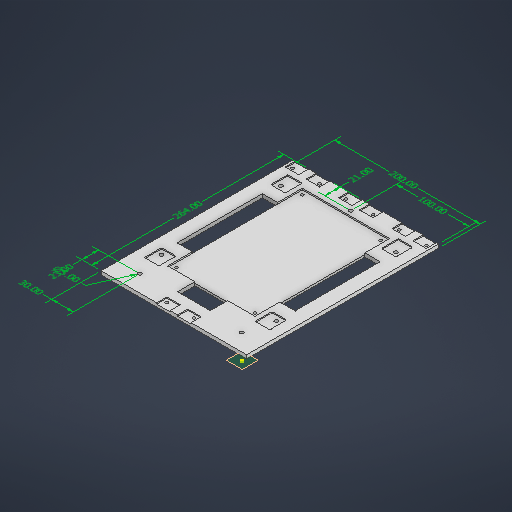
# Autodesk Inventor part: RobotPCBLevel
Saved by Autodesk Inventor 2026 (Build 300175000, 175)
## iProperties
Created: 2025-07-23
Part Number: RobotPCBLevel
Material: Generic
Document SubType Name: Modeling
Designer: jsmal
Density: 1 g/cm^3
Appearance: Default
Author: jsmal
Autodesk Inventor part; units mm, degrees
ref_plane "YZ Plane" through (0, 0, 0) normal (1, 0, 0) x (0, 1, 0)
ref_plane "XZ Plane" through (0, 0, 0) normal (0, 1, 0) x (-1, 0, 0)
ref_plane "XY Plane" through (0, 0, 0) normal (0, 0, 1) x (1, 0, 0)
sketch "Sketch1" plane through (0, 0, 0) normal (0, 1, 0) x (-1, 0, 0)
  point P0 (0, 0)
sketch "Sketch2" plane through (0, 0, 0) normal (0, 1, 0) x (-1, 0, 0)
  line L0 (0, 0) -> (200, 0)
  line L1 (200, 0) -> (200, -276)
  line L2 (200, -276) -> (0, -276)
  line L3 (0, -276) -> (0, 0)
  dimension "d0" = 200
  dimension "d1" = 276
  constraints: 8 end point, 2 parallel, 1 horizontal, 1 perpendicular
  measures "d0" distance of L1.end L2.end
  measures "d1" distance of L0.end L1.end
extrude "Extrusion1" add sketch "Sketch2" along normal blind 5
sketch "Sketch4" plane through (0, 5, 0) normal (0, 1, 0) x (1, 0, 0)
  line L0 (-40, 57.5) -> (-160, 57.5)
  line L1 (-160, 57.5) -> (-160, 242.5)
  line L2 (-160, 242.5) -> (-40, 242.5)
  line L3 (-40, 242.5) -> (-40, 57.5)
  line L4 (-200, 0) -> (0, 0) projected
  line L5 (0, 0) -> (0, 276) projected
  point P0 (-40, 150)
  dimension "d4" = 120
  dimension "d5" = 185
  dimension "d6" = 57.5
  dimension "d7" = 40
  constraints: 8 end point, 2 parallel, 1 horizontal, 1 midpoint, 1 perpendicular
  measures "d4" distance of L1.end L2.end
  measures "d5" distance of L0.end L1.end
  measures "d6" distance between parallel lines of L4 L0
  measures "d7" distance from line of L5 point (-40, 150)
extrude "Extrusion2" cut sketch "Sketch4" against normal blind 2
sketch "Sketch5" plane through (0, 3, 0) normal (0, 1, 0) x (1, 0, 0)
  line L0 (-40, 57.5) -> (-160, 57.5) projected
  line L1 (-160, 57.5) -> (-160, 242.5) projected
  line L2 (-160, 242.5) -> (-40, 242.5) projected
  line L3 (-40, 242.5) -> (-40, 57.5) projected
  point P0 (0, 0)
  point P1 (-154, 63.5)
  point P2 (-46, 63.5)
  point P3 (-154, 236.5)
  point P4 (-46, 236.5)
  dimension "d10" = 6
  dimension "d18" = 6
  dimension "d19" = 6
  dimension "d20" = 6
  dimension "d21" = 6
  dimension "d22" = 6
  dimension "d23" = 6
  dimension "d24" = 6
  measures "d10" distance from line of L0 point (-154, 63.5)
  measures "d18" distance from line of L1 point (-154, 63.5)
  measures "d19" distance from line of L1 point (-154, 236.5)
  measures "d20" distance from line of L2 point (-154, 236.5)
  measures "d21" distance from line of L2 point (-46, 236.5)
  measures "d22" distance from line of L3 point (-46, 236.5)
  measures "d23" distance from line of L3 point (-46, 63.5)
  measures "d24" distance from line of L0 point (-46, 63.5)
hole "Hole1" at (-154, 3, -63.5) at (-154, 3, -236.5) at (-46, 3, -236.5) at (-46, 3, -63.5) direction (0, -1, 0) diameter 4 depth 3 tip angle 118
sketch "Sketch6" plane through (0, 5, 0) normal (0, 1, 0) x (1, 0, 0)
  line L0 (-40, 57.5) -> (-160, 57.5) projected
  line L1 (-77.5, 57.5) -> (-122.5, 57.5)
  line L2 (-122.5, 57.5) -> (-122.5, 33.5)
  line L3 (-122.5, 33.5) -> (-77.5, 33.5)
  line L4 (-77.5, 33.5) -> (-77.5, 57.5)
  line L5 (-40, 242.5) -> (-40, 57.5) projected
  line L6 (-160, 57.5) -> (-160, 242.5) projected
  point P0 (0, 0)
  dimension "d25" = 45
  dimension "d26" = 24
  dimension "d27" = 37.5
  dimension "d28" = 37.5
  constraints: 8 end point, 2 parallel, 1 horizontal, 1 perpendicular, 1 point on line
  measures "d25" distance of L3.end L2.end
  measures "d26" distance of L2.end L1.end
  measures "d27" distance between parallel lines of L4 L5
  measures "d28" distance between parallel lines of L6 L2
extrude "Extrusion3" cut sketch "Sketch6" against normal blind 5
sketch "Sketch7" plane through (0, 5, 0) normal (0, 1, 0) x (1, 0, 0)
  line L0 (-40, 242.5) -> (-40, 57.5) projected
  line L1 (-40, 208.5) -> (-19, 208.5)
  line L2 (-19, 208.5) -> (-19, 91.5)
  line L3 (-19, 91.5) -> (-40, 91.5)
  line L4 (-40, 91.5) -> (-40, 208.5)
  line L5 (-160, 242.5) -> (-40, 242.5) projected
  line L6 (-160, 57.5) -> (-160, 242.5) projected
  line L7 (-160, 208.5) -> (-181, 208.5)
  line L8 (-181, 208.5) -> (-181, 91.5)
  line L9 (-181, 91.5) -> (-160, 91.5)
  line L10 (-160, 91.5) -> (-160, 208.5)
  point P0 (0, 0)
  dimension "d31" = 21
  dimension "d32" = 117
  dimension "d33" = 34
  dimension "d34" = 21
  dimension "d35" = 117
  dimension "d36" = 34
  constraints: 16 end point, 4 parallel, 2 horizontal, 2 perpendicular, 2 point on line
  measures "d31" distance of L2.end L3.end
  measures "d32" distance of L1.end L2.end
  measures "d33" distance between parallel lines of L5 L1
  measures "d34" distance of L9.end L8.end
  measures "d35" distance of L8.end L7.end
  measures "d36" distance between parallel lines of L5 L7
extrude "Extrusion4" cut sketch "Sketch7" against normal blind 5
sketch "Sketch8" plane through (0, 5, 0) normal (0, 1, 0) x (1, 0, 0)
  line L0 (0, 276) -> (-200, 276) projected
  line L1 (-3, 276) -> (-50.3, 276)
  line L2 (-50.3, 276) -> (-50.3, 256)
  line L3 (-50.3, 256) -> (-3, 256)
  line L4 (-3, 256) -> (-3, 276)
  line L5 (-76.35, 276) -> (-123.65, 276)
  line L6 (-123.65, 276) -> (-123.65, 256)
  line L7 (-123.65, 256) -> (-76.35, 256)
  line L8 (-76.35, 256) -> (-76.35, 276)
  line L9 (-149.7, 276) -> (-197, 276)
  line L10 (-197, 276) -> (-197, 256)
  line L11 (-197, 256) -> (-149.7, 256)
  line L12 (-149.7, 256) -> (-149.7, 276)
  line L13 (0, 0) -> (0, 276) projected
  line L14 (-200, 276) -> (-200, 0) projected
  line L15 (-3, 256) -> (-21.5, 256)
  line L16 (-21.5, 256) -> (-21.5, 276)
  line L17 (-21.5, 276) -> (-3, 276)
  line L18 (-3, 276) -> (-3, 256)
  line L19 (-50.3, 256) -> (-31.8, 256)
  line L20 (-31.8, 256) -> (-31.8, 276)
  line L21 (-31.8, 276) -> (-50.3, 276)
  line L22 (-50.3, 276) -> (-50.3, 256)
  line L23 (-76.35, 256) -> (-94.85, 256)
  line L24 (-94.85, 256) -> (-94.85, 276)
  line L25 (-94.85, 276) -> (-76.35, 276)
  line L26 (-76.35, 276) -> (-76.35, 256)
  line L27 (-123.65, 256) -> (-105.15, 256)
  line L28 (-105.15, 256) -> (-105.15, 276)
  line L29 (-105.15, 276) -> (-123.65, 276)
  line L30 (-123.65, 276) -> (-123.65, 256)
  line L31 (-149.7, 256) -> (-168.2, 256)
  line L32 (-168.2, 256) -> (-168.2, 276)
  line L33 (-168.2, 276) -> (-149.7, 276)
  line L34 (-149.7, 276) -> (-149.7, 256)
  line L35 (-197, 256) -> (-178.5, 256)
  line L36 (-178.5, 256) -> (-178.5, 276)
  line L37 (-178.5, 276) -> (-197, 276)
  line L38 (-197, 276) -> (-197, 256)
  point P0 (-3, 266)
  point P1 (-197, 266)
  dimension "d39" = 47.3
  dimension "d40" = 20
  dimension "d41" = 47.3
  dimension "d42" = 20
  dimension "d43" = 47.3
  dimension "d44" = 20
  dimension "d45" = 3
  dimension "d46" = 76.35
  dimension "d79" = 3
  dimension "d80" = 26.05
  dimension "d81" = 26.05
  dimension "d82" = 76.35
  dimension "d83" = 18.5
  dimension "d84" = 20
  dimension "d85" = 18.5
  dimension "d86" = 20
  dimension "d87" = 18.5
  dimension "d88" = 20
  dimension "d89" = 18.5
  dimension "d90" = 20
  dimension "d91" = 18.5
  dimension "d92" = 20
  dimension "d93" = 18.5
  dimension "d94" = 20
  constraints: 72 end point, 18 parallel, 9 horizontal, 9 perpendicular, 3 point on line, 2 midpoint
  measures "d39" distance of L3.end L2.end
  measures "d40" distance of L2.end L1.end
  measures "d41" distance of L7.end L6.end
  measures "d42" distance of L6.end L5.end
  measures "d43" distance of L11.end L10.end
  measures "d44" distance of L10.end L9.end
  measures "d45" distance from line of L13 point (-3, 266)
  measures "d46" distance between parallel lines of L13 L8
  measures "d79" distance between parallel lines of L14 L10
  measures "d80" distance between parallel lines of L6 L12
  measures "d81" distance between parallel lines of L2 L8
  measures "d82" distance between parallel lines of L14 L6
  measures "d83" distance of L16.end L17.end
  measures "d84" distance of L15.end L16.end
  measures "d85" distance of L21.end L20.end
  measures "d86" distance of L20.end L19.end
  measures "d87" distance of L24.end L25.end
  measures "d88" distance of L23.end L24.end
  measures "d89" distance of L29.end L28.end
  measures "d90" distance of L28.end L27.end
  measures "d91" distance of L32.end L33.end
  measures "d92" distance of L31.end L32.end
  measures "d93" distance of L37.end L36.end
  measures "d94" distance of L36.end L35.end
extrude "Extrusion5" cut sketch "Sketch8" against normal blind 1.5 contours L4 L3 L16 L0 | L20 L3 L2 L0 | L8 L7 L24 L0 | L28 L7 L6 L0 | L12 L11 L32 L0 | L36 L11 L10 L0
sketch "Sketch11" plane through (0, 3.5, 0) normal (0, 1, 0) x (1, 0, 0)
  line L0 (-3, 256) -> (-21.5, 256) projected
  line L1 (-3, 276) -> (-3, 256) projected
  line L2 (-31.8, 256) -> (-50.3, 256) projected
  line L3 (-50.3, 256) -> (-50.3, 276) projected
  line L4 (-76.35, 256) -> (-94.85, 256) projected
  line L5 (-76.35, 276) -> (-76.35, 256) projected
  line L6 (-105.15, 256) -> (-123.65, 256) projected
  line L7 (-123.65, 256) -> (-123.65, 276) projected
  line L8 (-149.7, 256) -> (-168.2, 256) projected
  line L9 (-149.7, 276) -> (-149.7, 256) projected
  line L10 (-178.5, 256) -> (-197, 256) projected
  line L11 (-197, 256) -> (-197, 276) projected
  point P0 (0, 0)
  point P1 (-192, 261)
  point P2 (-154.7, 261)
  point P3 (-118.65, 261)
  point P4 (-81.35, 261)
  point P5 (-45.3, 261)
  point P6 (-8, 261)
  dimension "d97" = 5
  dimension "d98" = 5
  dimension "d99" = 5
  dimension "d100" = 5
  dimension "d101" = 5
  dimension "d102" = 5
  dimension "d103" = 5
  dimension "d104" = 5
  dimension "d105" = 5
  dimension "d106" = 5
  dimension "d107" = 5
  dimension "d108" = 5
  measures "d97" distance from line of L0 point (-8, 261)
  measures "d98" distance from line of L1 point (-8, 261)
  measures "d99" distance from line of L2 point (-45.3, 261)
  measures "d100" distance from line of L3 point (-45.3, 261)
  measures "d101" distance from line of L4 point (-81.35, 261)
  measures "d102" distance from line of L5 point (-81.35, 261)
  measures "d103" distance from line of L6 point (-118.65, 261)
  measures "d104" distance from line of L7 point (-118.65, 261)
  measures "d105" distance from line of L8 point (-154.7, 261)
  measures "d106" distance from line of L9 point (-154.7, 261)
  measures "d107" distance from line of L10 point (-192, 261)
  measures "d108" distance from line of L11 point (-192, 261)
hole "Hole2" at (-8, 3.5, -261) at (-45.3, 3.5, -261) at (-81.35, 3.5, -261) at (-118.65, 3.5, -261) at (-154.7, 3.5, -261) at (-192, 3.5, -261) direction (0, -1, 0) diameter 4 depth 5 tip angle 118
sketch "Sketch12" plane through (0, 5, 0) normal (0, 1, 0) x (1, 0, 0)
  line L0 (-76.35, 0) -> (-123.65, 0)
  line L1 (-123.65, 0) -> (-123.65, 20)
  line L2 (-123.65, 20) -> (-76.35, 20)
  line L3 (-76.35, 20) -> (-76.35, 0)
  line L4 (0, 0) -> (0, 276) projected
  line L5 (-76.35, 0) -> (-94.85, 0)
  line L6 (-94.85, 0) -> (-94.85, 20)
  line L7 (-94.85, 20) -> (-76.35, 20)
  line L8 (-76.35, 20) -> (-76.35, 0)
  line L9 (-123.65, 20) -> (-105.15, 20)
  line L10 (-105.15, 20) -> (-105.15, 0)
  line L11 (-105.15, 0) -> (-123.65, 0)
  line L12 (-123.65, 0) -> (-123.65, 20)
  dimension "d116" = 47.3
  dimension "d117" = 20
  dimension "d118" = 76.35
  dimension "d119" = 18.5
  dimension "d120" = 20
  dimension "d121" = 18.5
  dimension "d122" = 20
  constraints: 24 end point, 6 parallel, 3 horizontal, 3 perpendicular
  measures "d116" distance of L1.end L2.end
  measures "d117" distance of L0.end L1.end
  measures "d118" distance between parallel lines of L4 L3
  measures "d119" distance of L6.end L7.end
  measures "d120" distance of L5.end L6.end
  measures "d121" distance of L10.end L11.end
  measures "d122" distance of L9.end L10.end
extrude "Extrusion6" cut sketch "Sketch12" against normal blind 1.5 contours L0 L6 L2 L3 | L0 L1 L2 L10
sketch "Sketch13" plane through (0, 3.5, 0) normal (0, 1, 0) x (1, 0, 0)
  line L0 (-76.35, 20) -> (-76.35, 0) projected
  line L1 (-94.85, 20) -> (-76.35, 20) projected
  line L2 (-123.65, 20) -> (-105.15, 20) projected
  line L3 (-123.65, 0) -> (-123.65, 20) projected
  point P0 (0, 0)
  point P1 (-81.35, 15)
  point P2 (-118.65, 15)
  dimension "d125" = 5
  dimension "d126" = 5
  dimension "d127" = 5
  dimension "d128" = 5
  measures "d125" distance from line of L0 point (-81.35, 15)
  measures "d126" distance from line of L1 point (-81.35, 15)
  measures "d127" distance from line of L2 point (-118.65, 15)
  measures "d128" distance from line of L3 point (-118.65, 15)
hole "Hole3" at (-81.35, 3.5, -15) at (-118.65, 3.5, -15) direction (0, -1, 0) diameter 4 depth 5 tip angle 118
sketch "Sketch14" plane through (0, 5, 0) normal (0, 1, 0) x (1, 0, 0)
  line L0 (-40, 242.5) -> (-40, 208.5) projected
  line L1 (-21.5, 276) -> (-31.8, 276) projected
  line L2 (-160, 242.5) -> (-40, 242.5) projected
  line L3 (-186, 248.5) -> (-186, 225)
  line L4 (-186, 225) -> (-166, 225)
  line L5 (-166, 225) -> (-166, 248.5)
  line L6 (-160, 208.5) -> (-160, 242.5) projected
  line L7 (-186, 75) -> (-166, 75)
  line L8 (-166, 75) -> (-166, 51.5)
  line L9 (-186, 51.5) -> (-186, 75)
  line L10 (-122.5, 57.5) -> (-160, 57.5) projected
  line L11 (-160, 57.5) -> (-160, 91.5) projected
  line L12 (-40, 91.5) -> (-40, 57.5) projected
  line L13 (-40, 57.5) -> (-77.5, 57.5) projected
  line L14 (-14, 75) -> (-34, 75)
  line L15 (-34, 75) -> (-34, 51.5)
  line L16 (-14, 51.5) -> (-14, 75)
  line L17 (-34, 248.5) -> (-34, 225)
  line L18 (-34, 225) -> (-14, 225)
  line L19 (-14, 225) -> (-14, 248.5)
  line L20 (-166, 248.5) -> (-186, 248.5)
  line L21 (-34, 248.5) -> (-14, 248.5)
  line L22 (-34, 51.5) -> (-14, 51.5)
  line L23 (-166, 51.5) -> (-186, 51.5)
  point P0 (0, 0)
  point P1 (-26.65, 276)
  point P2 (-166, 265)
  point P3 (-160, 248.5)
  point P4 (-160, 35)
  point P5 (-160, 51.5)
  point P6 (-40, 35)
  point P7 (-40, 248.5)
  point P8 (-40, 265)
  point P9 (-40, 225.5)
  dimension "d143" = 20
  dimension "d147" = 6
  dimension "d154" = 6
  dimension "d168" = 6
  dimension "d170" = 20
  dimension "d175" = 6
  constraints: 32 end point, 9 point on line, 5 perpendicular, 4 parallel, 3 horizontal, 2 midpoint
  measures "d143" distance of L4.end L3.end
  measures "d147" distance between parallel lines of L6 L5
  measures "d154" distance between parallel lines of L11 L8
  measures "d168" distance between parallel lines of L12 L15
  measures "d170" distance of L7.start L7.end
  measures "d175" distance from line of point (-40, 225.5) L17
extrude "Extrusion7" cut sketch "Sketch14" against normal blind 1.5
fillet "Fillet1" radius 2 12 edges at (-14, 4.25, -248.5) (-14, 4.25, -225) (-34, 4.25, -225) (-14, 4.25, -51.5) (-14, 4.25, -75) (-34, 4.25, -75) (-186, 4.25, -75) (-166, 4.25, -51.5) (-166, 4.25, -75) (-186, 4.25, -225) (-166, 4.25, -248.5) (-166, 4.25, -225)
sketch "Sketch15" plane through (0, 3.5, 0) normal (0, 1, 0) x (1, 0, 0)
  line L0 (-14, 246.5) -> (-14, 227) projected
  line L1 (-16, 225) -> (-32, 225) projected
  line L2 (-32, 75) -> (-16, 75) projected
  line L3 (-14, 73) -> (-14, 53.5) projected
  line L4 (-16, 35) -> (-52, 35) projected
  line L5 (-54, 37) -> (-54, 49.5) projected
  line L6 (-186, 51.5) -> (-186, 73) projected
  line L7 (-184, 75) -> (-168, 75) projected
  line L8 (-168, 225) -> (-184, 225) projected
  line L9 (-186, 227) -> (-186, 248.5) projected
  line L10 (-178.5, 265) -> (-148, 265) projected
  point P0 (0, 0)
  point P1 (-21, 232)
  point P2 (-16, 265)
  point P3 (-21, 68)
  point P4 (-179, 68)
  point P5 (-186, 37)
  point P6 (-179, 232)
  point P7 (-186, 263)
  point P8 (-184, 265)
  point P9 (-14, 256)
  point P10 (-186, 256)
  dimension "d180" = 7
  dimension "d181" = 7
  dimension "d184" = 7
  dimension "d185" = 7
  dimension "d194" = 7
  dimension "d195" = 7
  dimension "d196" = 7
  dimension "d197" = 7
  measures "d180" distance from line of L0 point (-21, 232)
  measures "d181" distance from line of L1 point (-21, 232)
  measures "d184" distance from line of L2 point (-21, 68)
  measures "d185" distance from line of L3 point (-21, 68)
  measures "d194" distance from line of L7 point (-179, 68)
  measures "d195" distance from line of L6 point (-179, 68)
  measures "d196" distance from line of L8 point (-179, 232)
  measures "d197" distance from line of L9 point (-179, 232)
hole "Hole4" at (-21, 3.5, -232) at (-21, 3.5, -68) at (-179, 3.5, -68) at (-179, 3.5, -232) direction (0, -1, 0) diameter 5 depth 5 tip angle 118
ref_plane "Work Plane1" through (0, 1.5, 0) normal (0, -1, 0) x (1, 0, 0)
sketch "Sketch18" plane through (0, 5, 0) normal (0, 1, 0) x (1, 0, 0)
  line L0 (0, 276) -> (-200, 276) projected
  line L1 (0, 0) -> (0, 276) projected
  line L2 (-200, 276) -> (0, 276)
  line L3 (0, 276) -> (0, 270)
  line L4 (0, 270) -> (-200, 270)
  line L5 (-200, 270) -> (-200, 276)
  dimension "d275" = 6
  constraints: 8 end point, 2 parallel, 1 horizontal, 1 perpendicular, 1 point on line
  measures "d275" distance of L2.end L3.end
extrude "Extrusion9" cut sketch "Sketch18" against normal blind 10
sketch "Sketch19" plane through (0, 5, 0) normal (0, 1, 0) x (1, 0, 0)
  line L0 (-200, 270) -> (-200, 0) projected
  line L1 (-200, 0) -> (0, 0)
  line L2 (0, 0) -> (0, 6)
  line L3 (0, 6) -> (-200, 6)
  line L4 (-200, 6) -> (-200, 0)
  dimension "d278" = 6
  constraints: 8 end point, 2 parallel, 1 horizontal, 1 perpendicular
  measures "d278" distance of L2.end L1.end
extrude "Extrusion10" cut sketch "Sketch19" against normal blind 10
sketch "Sketch20" plane through (0, 5, 0) normal (0, 1, 0) x (1, 0, 0)
  line L0 (-200, 270) -> (-200, 6) projected
  line L1 (-200, 6) -> (-123.65, 6) projected
  line L2 (-76.35, 6) -> (0, 6) projected
  line L3 (0, 6) -> (0, 270) projected
  line L4 (-94.85, 270) -> (-105.15, 270) projected
  point P0 (0, 0)
  point P1 (-170, 29)
  point P2 (-30, 29)
  point P3 (-100, 249)
  dimension "d281" = 30
  dimension "d289" = 23
  dimension "d290" = 23
  dimension "d291" = 30
  dimension "d292" = 21
  dimension "d293" = 100
  measures "d281" distance from line of L0 point (-170, 29)
  measures "d289" distance from line of L1 point (-170, 29)
  measures "d290" distance from line of L2 point (-30, 29)
  measures "d291" distance from line of L3 point (-30, 29)
  measures "d292" distance from line of L4 point (-100, 249)
  measures "d293" distance from line of L3 point (-100, 249)
hole "Hole6" at (-170, 5, -29) at (-30, 5, -29) at (-100, 5, -249) direction (0, -1, 0) diameter 5 depth 5 tip angle 118
body "Solid1"
